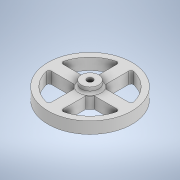
# Autodesk Inventor part: wheel
Saved by Autodesk Inventor 2021 (Build 250183000, 183)
## iProperties
Created: 2021-03-22
Part Number: wheel
Material: Generic
Document SubType Name: Modeling
Designer: awitc
Density: 1 g/cm^3
Appearance: Default
Author: awitc
Autodesk Inventor part; units mm, degrees
ref_plane "YZ Plane" through (0, 0, 0) normal (1, 0, 0) x (0, 1, 0)
ref_plane "XZ Plane" through (0, 0, 0) normal (0, 1, 0) x (-1, 0, 0)
ref_plane "XY Plane" through (0, 0, 0) normal (0, 0, 1) x (1, 0, 0)
sketch "Sketch5" plane through (0, 0, 0) normal (0, 1, 0) x (-1, 0, 0)
  circle A0 centre (0, 0) radius 2.55
  circle A1 centre (0, 0) radius 7.5
  circle A2 centre (0, 0) radius 36
  dimension "d10" = 5.1
  dimension "d11" = 15
  dimension "d12" = 72
  constraints: 3 centre point, 3 coincident
  measures "d10" diameter of A0
  measures "d11" diameter of A1
  measures "d12" diameter of A2
extrude "Extrusion4" add sketch "Sketch5" along normal blind 10 contours A2
extrude "Extrusion5" add sketch "Sketch5" along normal blind 15 contours A1
sketch "Sketch6" plane through (0, 0, 0) normal (0, -1, 0) x (1, 0, 0)
  circle A0 centre (0, 0) radius 10
  circle A1 centre (0, 0) radius 2.55 projected
  circle A2 centre (0, 0) radius 36
  circle A3 centre (0, 0) radius 2.55 projected
  circle A4 centre (0, 0) radius 31
  line L0 (-30.5941, 5) -> (-10, 5)
  line L1 (-30.5941, -5) -> (-10, -5)
  line L2 (-10, -5) -> (-8.6603, -5)
  line L3 (-10, 5) -> (-8.6603, 5)
  circle A5 centre (0, 0) radius 10
  line L4 (8.6603, -5) -> (30.5941, -5)
  line L5 (8.6603, 5) -> (30.5941, 5)
  line L6 (5, 10) -> (5, 30.5941)
  line L7 (5, 10) -> (5, 8.6603)
  line L8 (5, -8.6603) -> (5, -30.5941)
  line L9 (-5, 8.6603) -> (-5, 30.5941)
  line L10 (-5, -8.6603) -> (-5, -30.5941)
  dimension "d17" = 20
  constraints: 22 end point, 8 point on circle, 4 coincident, 3 centre point, 3 point on line, 2 horizontal, 2 parallel, 1 concentric, 1 vertical, 10 other
  measures "d17" diameter of A0
extrude "Extrusion6" cut sketch "Sketch6" against normal up to surface (10 mm away) contours A0 L7 L6 A4 L5 | L4 A4 L8 A0 | A0 L3 L0 A4 L9 | L10 A4 L1 L2 A0
fillet "Fillet1" radius 2 8 edges at (-5, 5, -30.5941) (-30.5941, 5, -5) (-30.5941, 5, 5) (-5, 5, 30.5941) (5, 5, 30.5941) (30.5941, 5, 5) (30.5941, 5, -5) (5, 5, -30.5941)
fillet "Fillet2" radius 2 1 edges at (7.5, 10, 0)
body "Solid2"
